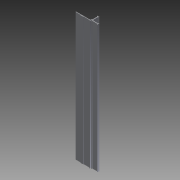
# Autodesk Inventor part: MayTec 1.19.19040_19 inch special profile, PG 40_329
Saved by Autodesk Inventor 2016 (Build 200138000, 138)
## iProperties
Category: PARTsolutions
Company: MAYTEC
Created: 2012-11-14
Part Number: MayTec 1.19.19040_19 inch special profile, PG 40_329
Catalog Web Link: www.cadenas.de
Description: 1.19.19040-19 inch special profile, PG 40
Vendor: MAYTEC
Document SubType Name: Modeling
Designer: PARTuser1
Manufacturer: MAYTEC
Density: 1 g/cm^3
Material: Generic
Appearance: RGB(175.94999939203154,175.94999939203154,175.94999939203154)
Mass: 49.397 g
Surface Area: 579.488 cm^2
Volume: 49.397 cm^3
PSOL_IDENT_0: {\\10.0.0.242\data_v9\23d-libs\maytec\maytec_3d\profile\zusatzprofile\19_zusatzprofile\1.19.19040.pr
PSOL_IDENT_1: j},251 {VTYP=3D},{NB=MayTec 1.19.19040_19 inch special profile, PG 40_329},{LINA=MayTec 1.19.19040_1
PSOL_IDENT_2: 9 inch special profile, PG 40_329},{NN=1.19.19040},{DATE=28.01.2010 09:42:17},{GEOMDATE=28.01.2010 0
PSOL_IDENT_3: 0:00:00},{VERSION=},{LINEID=10},{LINESUBID=-1},{WBVAR=L}  {NB=MayTec 1.19.19040_19 inch special prof
PSOL_IDENT_4: ile, PG 40_329},{LINA=MayTec 1.19.19040_19 inch special profile, PG 40_329},{KT=DUMMY},{PARTNR=1.19.
PSOL_IDENT_5: 19040},{DESCRIPTION=19 zoll Zusatzprofil, PG 40},{L=329.0},{XTRANS=19 inch special profile, PG 40}
CNS_NT: 19 inch special profile, PG 40
CNS_NB: MayTec 1.19.19040_19 inch special profile, PG 40_329
CNS_NBSYN: MayTec $PARTNR._$XTRANS._$L.
CNS_LINA: MayTec 1.19.19040_19 inch special profile, PG 40_329
CNS_PARTNR: 1.19.19040
CNS_DESCRIPTION: 19 inch special profile, PG 40
CNS_L: 329.0
CNS_XTRANS: 19 inch special profile, PG 40
SUPPLIER: MAYTEC
ARTICLENO: MayTec 1.19.19040_19 inch special profile, PG 40_329
BOMINFO: MayTec 1.19.19040_19 inch special profile, PG 40_329
CREATOR: CADENAS GmbH
Title: MayTec 1.19.19040_19 inch special profile, PG 40_329
Author: Cadenas PARTsolutions
Comments: 19 inch special profile, PG 40
Autodesk Inventor part; units mm, degrees
sketch "Skizze_1" plane through (0, 0, 0) normal (0, 0, 1) x (1, 0, 0)
  arc A0 (-39.4404, -19.0226) -> (-39.1984, -19.5) centre (-39.1984, -19.2) ccw
  line L0 (-39.1984, -19.5) -> (-26.5, -19.5)
  line L1 (-26.5, -19.5) -> (-26.5, -20.5)
  line L2 (-26.5, -20.5) -> (-18.5, -20.5)
  line L3 (-18.5, -20.5) -> (-18.5, -19.5)
  line L4 (-18.5, -19.5) -> (-2.5, -19.5)
  line L5 (-2.5, -19.5) -> (-2.5, -21)
  line L6 (-2.5, -21) -> (-1, -21)
  line L7 (-1, -21) -> (-1, -16)
  line L8 (-1, -16) -> (1, -16)
  line L9 (1, -16) -> (1, -19.5)
  line L10 (1, -19.5) -> (2.5, -19.5)
  line L11 (2.5, -19.5) -> (2.5, -18)
  line L12 (2.5, -18) -> (15.5, -18)
  line L13 (15.5, -18) -> (15.5, -19.5)
  line L14 (15.5, -19.5) -> (17, -19.5)
  line L15 (17, -19.5) -> (17, -14.5)
  line L16 (17, -14.5) -> (15.5, -14.5)
  line L17 (15.5, -14.5) -> (15.5, -16)
  line L18 (15.5, -16) -> (2.5, -16)
  line L19 (2.5, -16) -> (2.5, -14.5)
  line L20 (2.5, -14.5) -> (1, -14.5)
  line L21 (1, -14.5) -> (1, -1.5)
  line L22 (1, -1.5) -> (2.5, -1.5)
  line L23 (2.5, -1.5) -> (2.5, 0)
  line L24 (2.5, 0) -> (-2.5, 0)
  line L25 (-2.5, 0) -> (-2.5, -1.5)
  line L26 (-2.5, -1.5) -> (-1, -1.5)
  line L27 (-1, -1.5) -> (-1, -14.5)
  line L28 (-1, -14.5) -> (-2.5, -14.5)
  line L29 (-2.5, -14.5) -> (-2.5, -18)
  line L30 (-2.5, -18) -> (-38.4177, -18)
  line L31 (-38.4177, -18) -> (-39.4404, -19.0226)
  constraints: 64 end point, 2 point on circle, 1 centre point
extrude "Extrusion1" add sketch "Skizze_1" against normal blind 329
ref_plane "start_XY" through (-22.5, -19.5, 0) normal (0, 0, 1) x (1, 0, 0)
ref_plane "start_YZ" through (-22.5, -19.5, 0) normal (1, 0, 0) x (0, 1, 0)
ref_plane "start_ZX" through (-22.5, -19.5, 0) normal (0, 1, 0) x (0, 0, 1)
ref_plane "end_XY" through (-22.5, -19.5, -329) normal (0, 0, -1) x (1, 0, 0)
ref_plane "end_YZ" through (-22.5, -19.5, -329) normal (1, 0, 0) x (0, -1, 0)
ref_plane "end_ZX" through (-22.5, -19.5, -329) normal (0, -1, 0) x (0, 0, -1)
ref_plane "side_1a_XY" through (9, -16, -164.5) normal (0, 1, 0) x (1, 0, 0)
ref_plane "side_1a_YZ" through (9, -16, -164.5) normal (1, 0, 0) x (0, 0, -1)
ref_plane "side_1a_ZX" through (9, -16, -164.5) normal (0, 0, -1) x (0, 1, 0)
ref_plane "side_1b_XY" through (0, -16, -164.5) normal (0, -1, 0) x (-1, 0, 0)
ref_plane "side_1b_YZ" through (0, -16, -164.5) normal (-1, 0, 0) x (0, 0, -1)
ref_plane "side_1b_ZX" through (0, -16, -164.5) normal (0, 0, -1) x (0, -1, 0)
ref_plane "side_1_XY" through (-22.5, -18, -164.5) normal (0, 1, 0) x (1, 0, 0)
ref_plane "side_1_YZ" through (-22.5, -18, -164.5) normal (1, 0, 0) x (0, 0, -1)
ref_plane "side_1_ZX" through (-22.5, -18, -164.5) normal (0, 0, -1) x (0, 1, 0)
ref_plane "side_6a_XY" through (9, -18, -164.5) normal (0, -1, 0) x (-1, 0, 0)
ref_plane "side_6a_YZ" through (9, -18, -164.5) normal (-1, 0, 0) x (0, 0, -1)
ref_plane "side_6a_ZX" through (9, -18, -164.5) normal (0, 0, -1) x (0, -1, 0)
ref_plane "side_2_XY" through (-1, -8, -164.5) normal (-1, 0, 0) x (0, 1, 0)
ref_plane "side_2_YZ" through (-1, -8, -164.5) normal (0, 1, 0) x (0, 0, -1)
ref_plane "side_2_ZX" through (-1, -8, -164.5) normal (0, 0, -1) x (-1, 0, 0)
ref_plane "side_5_XY" through (1, -8, -164.5) normal (1, 0, 0) x (0, -1, 0)
ref_plane "side_5_YZ" through (1, -8, -164.5) normal (0, -1, 0) x (0, 0, -1)
ref_plane "side_5_ZX" through (1, -8, -164.5) normal (0, 0, -1) x (1, 0, 0)
ref_plane "side_6_XY" through (-22.5, -19.5, -164.5) normal (0, -1, 0) x (-1, 0, 0)
ref_plane "side_6_YZ" through (-22.5, -19.5, -164.5) normal (-1, 0, 0) x (0, 0, -1)
ref_plane "side_6_ZX" through (-22.5, -19.5, -164.5) normal (0, 0, -1) x (0, -1, 0)
body "Solid1"
